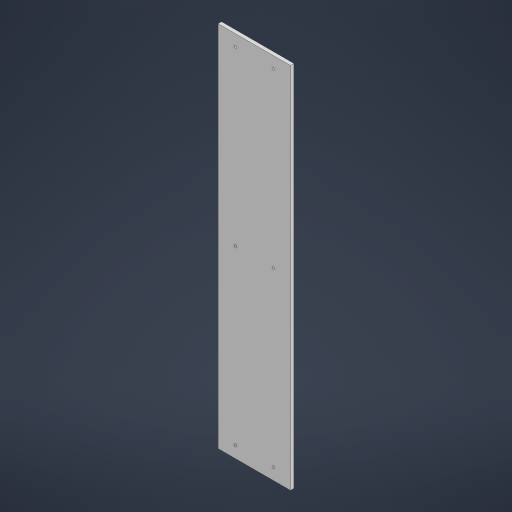
# Autodesk Inventor part: 10_outerlegg_short_side
Saved by Autodesk Inventor 2024 (Build 280153000, 153)
## iProperties
Created: 2023-05-24
Part Number: 10_outerlegg_short_side
Material: Generic
Document SubType Name: Modeling
Designer: aasmu
Density: 1 g/cm^3
Appearance: Default
outerlegg_plate_width: 6.000 mm
Author: aasmu
Autodesk Inventor part; units mm, degrees
ref_plane "YZ Plane" through (0, 0, 0) normal (1, 0, 0) x (0, 1, 0)
ref_plane "XZ Plane" through (0, 0, 0) normal (0, 1, 0) x (-1, 0, 0)
ref_plane "XY Plane" through (0, 0, 0) normal (0, 0, 1) x (1, 0, 0)
sketch "Sketch1" plane through (0, 0, 0) normal (0, 0, 1) x (1, 0, 0)
  line L0 (0, 0) -> (126, 0)
  line L1 (126, 0) -> (126, 640)
  line L2 (126, 640) -> (0, 640)
  line L3 (0, 640) -> (0, 0)
  line L4 (0, 40) -> (126, 40) construction
  circle A0 centre (30, 20) radius 2
  circle A1 centre (96, 20) radius 2
  line L5 (30, 40) -> (30, 0) construction
  line L6 (96, 20) -> (126, 20) construction
  line L7 (30, 20) -> (0, 20) construction
  line L8 (0, 320) -> (30, 320) construction
  line L9 (96, 320) -> (126, 320) construction
  circle A2 centre (30, 320) radius 2
  circle A3 centre (96, 320) radius 2
  circle A4 centre (30, 620) radius 2
  circle A5 centre (96, 620) radius 2
  dimension "d0" = 126
  dimension "d1" = 640
  dimension "d2" = 40
  dimension "d3" = 4
  dimension "d4" = 30
  constraints: 20 end point, 7 point on line, 6 centre point, 4 horizontal, 3 equal length, 3 equal radius, 3 midpoint, 3 perpendicular, 2 coincident, 2 parallel, 2 symmetric about line, 1 collinear, 2 other
  measures "d0" distance of L2.end L1.end
  measures "d1" distance of L1.end L0.end
  measures "d2" distance between parallel lines of L0 L4
  measures "d3" diameter of A0
  measures "d4" distance of L5.end L0.start
extrude "Extrusion1" add sketch "Sketch1" along normal blind 6
equation "\"d0\" = outer_carriage_length"
equation "\"d1\" = outerlegg_height"
equation "\"d2\" = outer_carriage_height"
equation "\"d3\" = outer_carriage_screw_size"
equation "\"d4\" = outer_carriage_corner_to_screw"
equation "\"d5\" = outerlegg_plate_width"
equation "\"outerlegg_plate_width\" = 6"
equation "\"outer_carriage_length\" = 126"
equation "\"outerlegg_height\" = 640"
equation "\"outer_carriage_height\" = 40"
equation "\"outer_carriage_screw_size\" = 4"
equation "\"outer_carriage_corner_to_screw\" = 30"
body "Solid1"
